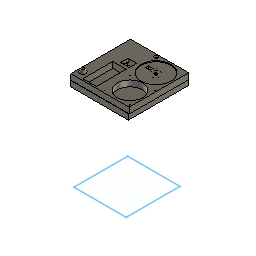
Untitled (1) (Autodesk Fusion 360 design; units mm, degrees)
part number: 2025-10-25-14-32-45-415
Autodesk Fusion 360 part; units mm, degrees
note: some values were not read from the file. Chosen so that the rebuilt part matches the saved one: which bodies a step acts on; which face or edge a step refers to. Set by a fixed rule: which sketch regions a step uses; the direction of a hole.
sketch "Sketch1" plane through (0, 0, 0) normal (0, 0, 1) x (1, 0, 0)
sketch "Sketch2" plane through (0, 0, 0) normal (0, 0, 1) x (1, 0, 0)
  line L0 (-50, 50) -> (50, 50)
  line L1 (50, 50) -> (50, -50)
  line L2 (50, -50) -> (-50, -50)
  line L3 (-50, -50) -> (-50, 50)
  line L4 (-40, 40) -> (40, 40)
  line L5 (40, 40) -> (40, -40)
  line L6 (40, -40) -> (-40, -40)
  line L7 (-40, -40) -> (-40, 40)
  line L8 (-50, -50) -> (50, -50)
  line L9 (50, -50) -> (50, 50)
  line L10 (50, 50) -> (-50, 50)
  line L11 (-50, 50) -> (-50, -50)
  line L12 (50, -50) -> (0, -50)
  constraint horizontal L0
  constraint vertical L1
  constraint vertical L3
  constraint horizontal L4
  constraint vertical L5
  constraint horizontal L6
  constraint vertical L7
  constraint vertical L9
  constraint horizontal L10
  constraint vertical L11
sketch "Sketch3" plane through (0, 0, 10) normal (0, 0, 1) x (-1, 0, 0)
  line L0 (40, 40) -> (-40, 40)
  line L1 (-40, 40) -> (-40, -40)
  line L2 (-40, -40) -> (40, -40)
  line L3 (40, -40) -> (40, 40)
  line L4 (50, -50) -> (-50, -50)
  line L5 (-50, -50) -> (-50, 50)
  line L6 (-50, 50) -> (50, 50)
  line L7 (50, 50) -> (50, -50)
  constraint horizontal L4
  constraint vertical L5
  constraint horizontal L6
  constraint vertical L7
sketch "Sketch4" plane through (50, 0, 0) normal (1, 0, 0) x (0, 1, 0)
  line L0 (-50, 10) -> (50, 10)
  line L1 (50, 10) -> (50, 60)
  line L2 (50, 60) -> (-50, 60)
  line L3 (-50, 60) -> (-50, 10)
  circle A0 centre (0, 20) radius 5
  dimension "d5" = 10
  measures "d5" diameter of A0
sketch "Sketch8" plane through (0, 0, 0) normal (0, 0, 1) x (1, 0, 0)
  line L0 (-99.8621, 99.5976) -> (95.1379, 99.5976)
  line L1 (95.1379, 99.5976) -> (95.1379, -100.4024)
  line L2 (95.1379, -100.4024) -> (-99.8621, -100.4024)
  line L3 (-99.8621, -100.4024) -> (-99.8621, 99.5976)
  circle A0 centre (40.1379, 44.5976) radius 49.5
  circle A1 centre (47.5, -50) radius 42.5
  circle A2 centre (47.5, -50) radius 22.5
  circle A3 through (0.1806, 90, 0.1954) (-7.3194, 94.3301, 0.1954) (-7.3194, 85.6699, 0.1954)
  arc A4 through (36.1908, 50.2562, 8.3931) (20.1221, 75.3764, 7.5452) (-4.8194, 90, 0.1954)
  circle A5 centre (40.1379, 44.5976) radius 15
  line L4 (-65, 5) -> (-20, 5)
  line L5 (-20, 5) -> (-20, -95)
  line L6 (-20, -95) -> (-65, -95)
  line L7 (-65, -95) -> (-65, 5)
  line L8 (-50, 40) -> (-20, 40)
  line L9 (-20, 40) -> (-20, 15)
  line L10 (-20, 15) -> (-50, 15)
  line L11 (-50, 15) -> (-50, 40)
  circle A6 centre (-50, 27.5) radius 12.5
  circle A7 centre (-85, -75) radius 10
  circle A8 centre (-85, -75) radius 5
  dimension "d42" = 60
  dimension "d43" = 55
  dimension "d44" = 55
  dimension "d45" = 99
  dimension "d46" = 10
  dimension "d47" = 30
  constraint horizontal L0
  constraint vertical L1
  constraint horizontal L2
  constraint vertical L3
  constraint concentric A1 A2
  constraint concentric A0 A5
  constraint horizontal L4
  constraint vertical L5
  constraint horizontal L6
  constraint vertical L7
  constraint horizontal L8
  constraint vertical L9
  constraint horizontal L10
  constraint vertical L11
  constraint coincident L10.end A6
  constraint tangent L10 A6
  constraint coincident L8.start A6
  constraint concentric A7 A8
  measures "d42" distance of origin A0.centre
  measures "d43" distance of L1 A0.centre
  measures "d44" distance of L0 A0.centre
  measures "d45" diameter of A0
  measures "d47" diameter of A5
extrude "Extrude6" add sketch "Sketch8" against normal blind 50 contours L0 L1 L2 L3 makes body 1
extrude "Extrude7" add sketch "Sketch8" along normal blind -2 and the other way blind 50 contours A1 bodies 1
extrude "Extrude8" add sketch "Sketch8" against normal blind 40 contours A2 bodies 1
extrude "Extrude9" cut sketch "Sketch8" against normal blind 5 contours A2 bodies 1
extrude "Extrude10" add sketch "Sketch8" against normal blind 5 contours A2 bodies 1
extrude "Extrude11" cut sketch "Sketch8" against normal blind 1 contours A2 bodies 1
fillet "Fillet1" radius 1 2 edges at (26.5226, -58.1363, -2) (26.5226, -41.8637, -1) on bodies 1
extrude "Extrude12" add sketch "Sketch8" along normal blind -3 and the other way blind 50 contours A0 bodies 1
sketch "Sketch9" plane through (0, 0, 0.1954) normal (0, 0, 1) x (1, 0, 0)
sketch "Sketch8 (curves 0.1954 mm off its plane)" plane through (0, 0, 0.1954) normal (0, 0, 1) x (1, 0, 0)
  circle A0 centre (-4.8194, 90) radius 5
extrude "Extrude13" add sketch "Sketch8 (curves 0.1954 mm off its plane)" along normal blind -50 and the other way blind -2 bodies 1
extrude "Extrude14" add sketch "Sketch8" against normal blind 50 contours A5 bodies 1
pipe "Pipe1" add diameter 1.25 path "Sketch8" along A4 bodies 1
extrude "Extrude15" add sketch "Sketch8" along normal blind 5 and the other way blind 50 contours L4 L5 L6 L7 bodies 1
extrude "Extrude16" add sketch "Sketch8" against normal blind 50 contours A7 bodies 1
extrude "Extrude17" add sketch "Sketch8" against normal blind 50 contours A8 bodies 1
sketch "Sketch10" plane through (0, 0, 0) normal (0, 0, 1) x (1, 0, 0)
  circle A0 through (-80, -75, 9) (-87.5, -70.6699, 9) (-87.5, -79.3301, 9)
sketch "Sketch10 (curves 9 mm off its plane)" plane through (0, 0, 9) normal (0, 0, 1) x (1, 0, 0)
  circle A0 centre (-85, -75) radius 5
loft "Loft1" add profiles "Sketch8", "Sketch10 (curves 9 mm off its plane)" section 1 contours A7 section 2 bodies 1
extrude "Extrude18" add sketch "Sketch8" against normal blind 50 contours L11 A6 | L8 L9 L10 A6 | L11 A6 bodies 1
extrude "Extrude19" add sketch "Sketch8" along normal blind 3 contours L8 L9 L10 A6 bodies 1
extrude "Extrude20" add sketch "Sketch8" against normal blind 50 contours A2 bodies 1
sketch "Sketch11" plane through (0, 0, 0) normal (0, 0, 1) x (1, 0, 0)
  line L0 (-110, 110) -> (110, 110)
  line L1 (110, 110) -> (110, -110)
  line L2 (110, -110) -> (-110, -110)
  line L3 (-110, -110) -> (-110, 110)
  constraint horizontal L0
  constraint vertical L1
  constraint horizontal L2
  constraint vertical L3
move_body "Move1" bodies 1 to x (1, 0, 0) y (0, 1, 0) z (0, 0, 1) at (0, 0, -60)
extrude "Extrude21" add sketch "Sketch11" against normal blind 10 separate body makes body 2
move_body "Move2" bodies 1 to x (1, 0, 0) y (0, 1, 0) z (0, 0, 1) at (0, 0, 80)
combine "Combine1" operation cut target body 1 tool bodies 2 makes body 3 at (-34.8621, 32.931, -30)
hole "Hole1" at (91.7266, 96.0315, -30) direction (0, 0, 1) diameter 2.53 depth 30 tip angle 118 bodies 1 3
thread "Thread1" "ISO Metric profile 3.0 M3x0.5 M3x0.5 6H" thread offset 0 thread depth 7.4
hole "Hole2" at (91.9072, -97.0072, -30) direction (0, 0, 1) diameter 2.53 depth 25 tip angle 118 bodies 3
thread "Thread2" "ISO Metric profile 3.0 M3x0.5 M3x0.5 6H" thread offset 0 thread depth 7.4
hole "Hole3" at (-94.6479, 94.5231, -30) direction (0, 0, 1) diameter 2.53 depth 30 tip angle 118 bodies 1 3
thread "Thread3" "ISO Metric profile 3.0 M3x0.5 M3x0.5 6H" thread offset 0 thread depth 7.4
hole "Hole4" at (-94.624, -94.9374, -30) direction (0, 0, 1) diameter 2.53 depth 30 tip angle 118 bodies 1 3
thread "Thread4" "ISO Metric profile 3.0 M3x0.5 M3x0.5 6H" thread offset 0 thread depth 7.4
move_body "Move3" bodies 3 to x (1, 0, 0) y (0, 1, 0) z (0, 0, 1) at (180, 0, -100)
move_body "Move4" bodies 3 to x (1, 0, 0) y (0, 1, 0) z (0, 0, 1) at (15, -205, 0)
sketch "Sketch12" plane through (0, 0, -110) normal (0, 0, 1) x (-1, 0, 0)
  circle A0 centre (-100.376, 299.9374) radius 1.2645
  circle A1 centre (-100.3521, 110.4769) radius 1.2645
  circle A2 centre (-286.9072, 302.0072) radius 1.2645
  circle A3 centre (-286.7266, 108.9685) radius 1.2645
  line L0 (-290.1379, 305.4024) -> (-290.1379, 105.4024)
  line L1 (-290.1379, 105.4024) -> (-95.1379, 105.4024)
  line L2 (-95.1379, 105.4024) -> (-95.1379, 305.4024)
  line L3 (-95.1379, 305.4024) -> (-290.1379, 305.4024)
  line L4 (-280, 295) -> (-105, 295)
  line L5 (-105, 295) -> (-105, 115)
  line L6 (-105, 115) -> (-280, 115)
  line L7 (-280, 115) -> (-280, 295)
  constraint horizontal L4
  constraint vertical L5
  constraint horizontal L6
  constraint vertical L7
extrude "Extrude22" cut sketch "Sketch12" against normal blind 15 contours L4 L5 L6 L7 bodies 3
extrude "Extrude23" cut sketch "Sketch8" along normal blind 20 and the other way blind -17 contours A5 bodies 1
hole "Hole5" at (40.1379, 44.5976, 0) direction (0, 0, 1) diameter 10 depth 25 tip angle 180 bodies 1
extrude "Extrude24" cut sketch "Sketch8" along normal blind 15 contours A5 bodies 1
extrude "Extrude25" cut sketch "Sketch8" along normal blind 20 contours A1 | A2 bodies 1
sketch "Sketch13" plane through (0, 0, 20) normal (0, 0, 1) x (-1, 0, 0)
  arc A0 (50, -15) -> (50, -40) centre (50, -27.5) ccw
  line L0 (50, -40) -> (20, -40)
  line L1 (20, -40) -> (20, -15)
  line L2 (20, -15) -> (50, -15)
  circle A1 centre (85, 75) radius 10
  circle A2 centre (4.8194, -90) radius 5
  circle A3 centre (-40.1379, -44.5976) radius 49.5
  line L3 (20, 95) -> (65, 95)
  line L4 (65, 95) -> (65, -5)
  line L5 (65, -5) -> (20, -5)
  line L6 (20, -5) -> (20, 95)
  circle A4 centre (-47.5, 50) radius 42.5
  line L7 (99.8621, 100.4024) -> (-95.1379, 100.4024)
  line L8 (-95.1379, 100.4024) -> (-95.1379, -99.5976)
  line L9 (-95.1379, -99.5976) -> (99.8621, -99.5976)
  line L10 (99.8621, -99.5976) -> (99.8621, 100.4024)
  line L11 (-47.5, 50) -> (-47.5, 92.5)
  line L12 (-47.5, 50) -> (-90, 50)
  line L13 (-90, 92.5) -> (-47.5, 92.5)
  line L14 (-90, 92.5) -> (-90, 50)
  line L15 (-5, 92.5) -> (-5, 50)
  line L16 (-5, 92.5) -> (-47.5, 92.5)
  line L17 (-90, 7.5) -> (-90, 50)
  line L18 (-90, 7.5) -> (-47.5, 7.5)
  line L19 (-5, 7.5) -> (-47.5, 7.5)
  line L20 (-5, 7.5) -> (-5, 50)
  constraint coincident A4.centre L11.start
  constraint coincident A4 L11.end
  constraint vertical L11
  constraint coincident A4 L12.end
  constraint perpendicular L11 L12
  constraint tangent A4 L13
  constraint tangent A4 L14
  constraint symmetric L13.end L11 L16.end
  constraint symmetric L11 L12.end L15.end
  constraint symmetric L11 L13.start L15.start
  constraint symmetric L11.end L12 L18.end
  constraint symmetric L14.end L12 L17.end
  constraint symmetric L12 L13.start L17.start
  constraint symmetric L12 L15.start L19.start
  constraint symmetric L12 L15.end L20.end
  constraint symmetric L12 L11.end L18.end
hole "Hole6" at (90, -92.5, 20) direction (0, 0, -1) diameter 2.53 depth 3 tip angle 118 bodies 1
thread "Thread5" "ISO Metric profile 3.0 M3x0.5 M3x0.5 6H" thread offset 0 thread depth 7.4
hole "Hole7" at (90, -7.5, 20) direction (0, 0, -1) diameter 2.53 depth 3 tip angle 118 bodies 1
thread "Thread6" "ISO Metric profile 3.0 M3x0.5 M3x0.5 6H" thread offset 0 thread depth 7.4
hole "Hole8" at (5, -7.5, 20) direction (0, 0, -1) diameter 2.53 depth 3 tip angle 118 bodies 1
thread "Thread7" "ISO Metric profile 3.0 M3x0.5 M3x0.5 6H" thread offset 0 thread depth 7.4
hole "Hole9" at (5, -92.5, 20) direction (0, 0, -1) diameter 2.53 depth 3 tip angle 118 bodies 1
thread "Thread8" "ISO Metric profile 3.0 M3x0.5 M3x0.5 6H" thread offset 0 thread depth 7.4
extrude "Extrude26" cut 1 faces at (-50, -61.6667, 25) along direction (0, 0, -1) blind 30 on bodies 1 bodies 1
extrude "Extrude27" cut sketch "Sketch8" along normal blind 20 contours A7 | A8 bodies 1
extrude "Extrude28" cut sketch "Sketch8" along normal blind 22 contours A8 bodies 1
extrude "Extrude29" cut 1 faces at (-25.845, 27.8114, 23) along direction (0, 0, -1) blind 40 on bodies 1 bodies 1
extrude "Extrude30" cut sketch "Sketch8" along normal blind 19 contours L11 A6 picked at (-47.7473, 31.0052) bodies 1
sketch "Sketch14" plane through (0, 0, 17) normal (0, 0, 1) x (-1, 0, 0)
  circle A0 centre (-40.1379, -44.5976) radius 5
  circle A1 centre (-40.1379, -44.5976) radius 49.5
  line L0 (-20, -55) -> (-5, -55)
  line L1 (-5, -55) -> (-5, -45)
  line L2 (-5, -45) -> (-20, -45)
  line L3 (-20, -45) -> (-20, -55)
  constraint horizontal L0
  constraint vertical L1
  constraint horizontal L2
  constraint vertical L3
extrude "Extrude31" cut sketch "Sketch14" against normal blind 37 contours L0 L1 L2 L3 bodies 1
move_body "Move5" bodies 3 to x (1, 0, 0) y (0, 1, 0) z (0, 0, 1) at (-308.4862, 306.1948, 0)
move_body "Move6" bodies 3 to x (1, 0, 0) y (0, 1, 0) z (0, 0, 1) at (110, -100, 110)
